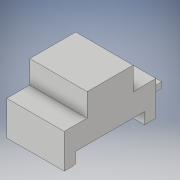
# Autodesk Inventor part: Model Creation 1
Saved by Autodesk Inventor 2019 (Build 230136000, 136)
## iProperties
Created: 2019-09-09
Part Number: Model Creation 1
Material: Generic
Document SubType Name: Modeling
Designer: IED8
Density: 1 g/cm^3
Appearance: Default
Author: IED8
Autodesk Inventor part; units mm, degrees
ref_plane "YZ Plane" through (0, 0, 0) normal (1, 0, 0) x (0, 1, 0)
ref_plane "XZ Plane" through (0, 0, 0) normal (0, 1, 0) x (-1, 0, 0)
ref_plane "XY Plane" through (0, 0, 0) normal (0, 0, 1) x (1, 0, 0)
sketch "Sketch1" plane through (0, 0, 0) normal (1, 0, 0) x (0, 1, 0)
  line L0 (0, 11.4777) -> (0, -1.2223)
  line L1 (0, -1.2223) -> (12.7, -1.2223)
  line L2 (12.7, -1.2223) -> (12.7, -77.4223)
  line L3 (12.7, -77.4223) -> (0, -77.4223)
  line L4 (0, -77.4223) -> (0, -90.1223)
  line L5 (0, -90.1223) -> (38.1, -90.1223)
  line L6 (38.1, -90.1223) -> (38.1, -64.7223)
  line L7 (38.1, -64.7223) -> (63.5, -64.7223)
  line L8 (63.5, -64.7223) -> (63.5, -13.9223)
  line L9 (63.5, -13.9223) -> (38.1, -13.9223)
  line L10 (38.1, -13.9223) -> (38.1, 11.4777)
  line L11 (38.1, 11.4777) -> (0, 11.4777)
  point P0 (0, 0)
  dimension "d0" = 12.7
  dimension "d1" = 12.7
  dimension "d2" = 76.2
  dimension "d3" = 12.7
  dimension "d4" = 38.1
  dimension "d5" = 25.4
  dimension "d6" = 25.4
  dimension "d7" = 50.8
  dimension "d8" = 25.4
  dimension "d9" = 25.4
  constraints: 24 end point, 6 perpendicular, 4 point on line, 1 parallel, 1 vertical
  measures "d0" distance of L0.start L0.end
  measures "d1" distance of L0.end L1.end
  measures "d2" distance of L1.end L2.end
  measures "d3" distance of L3.end L4.end
  measures "d4" distance of L4.end L5.end
  measures "d5" distance of L5.end L6.end
  measures "d6" distance of L6.end L7.end
  measures "d7" distance of L7.end L8.end
  measures "d8" distance of L8.end L9.end
  measures "d9" distance of L9.end L10.end
extrude "Extrusion1" add sketch "Sketch1" along normal blind 63.5
sketch "Sketch2" plane through (63.5, 0, 0) normal (1, 0, 0) x (0, 0, -1)
  point P0 (0, 0)
sketch "Sketch3" plane through (0, 0, -90.1223) normal (0, 0, -1) x (-1, 0, 0)
  line L0 (0, 38.1) -> (-63.5, 38.1) projected
  line L1 (-63.5, 38.1) -> (-63.5, 19.05)
  line L2 (-63.5, 0) -> (-63.5, 38.1) projected
  line L3 (-50.8, 19.05) -> (-12.7, 19.05)
  line L4 (-12.7, 19.05) -> (-12.7, 12.7)
  line L5 (0, 12.7) -> (-63.5, 12.7) projected
  line L6 (-12.7, 12.7) -> (-50.8, 12.7)
  line L7 (-50.8, 19.05) -> (-50.8, 12.7)
  point P0 (0, 0)
  dimension "d12" = 19.05
  dimension "d13" = 12.7
  dimension "d14" = 38.1
  dimension "d15" = 6.35
  constraints: 10 end point, 2 point on line, 1 midpoint, 1 perpendicular
  measures "d12" distance of L0.end L1.end
  measures "d13" distance of L1.end L3.start
  measures "d14" distance of L3.start L3.end
  measures "d15" distance of L3.end L4.end
extrude "Extrusion2" add sketch "Sketch3" along normal blind 19.05
body "Solid1"
